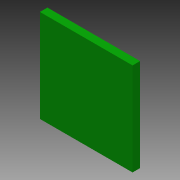
# Autodesk Inventor part: DisceepXL_PCB
Saved by Autodesk Inventor 2014 (Build 180170000, 170)
## iProperties
Created: 2014-11-22
Part Number: DisceepXL_PCB
Material: Phenolic Resin
Document SubType Name: Modeling
Designer: DV
Mass: 0.0449256 g
Surface Area: 1.26194 cm^2
Volume: 0.0325548 cm^3
Density: 1.38 g/cm^3
Appearance: Smooth - Light Orange
Author: DV
Autodesk Inventor part; units mm, degrees
ref_plane "YZ Plane" through (0, 0, 0) normal (1, 0, 0) x (0, 1, 0)
ref_plane "XZ Plane" through (0, 0, 0) normal (0, 1, 0) x (-1, 0, 0)
ref_plane "XY Plane" through (0, 0, 0) normal (0, 0, 1) x (1, 0, 0)
sketch "Sketch1" plane through (0, 0, 0) normal (0, 0, 1) x (1, 0, 0)
  line L0 (-3.683, -3.683) -> (3.683, -3.683)
  line L1 (3.683, -3.683) -> (3.683, 3.683)
  line L2 (3.683, 3.683) -> (-3.683, 3.683)
  line L3 (-3.683, 3.683) -> (-3.683, -3.683)
  point P0 (0, 0)
  dimension "d0" = 7.366
  dimension "d1" = 7.366
  dimension "d4" = 3.683
  dimension "d5" = 3.683
  constraints: 8 end point, 2 parallel, 1 horizontal, 1 perpendicular
  measures "d0" distance of L2.end L1.end
  measures "d1" distance of L1.end L0.end
  measures "d4" distance from line of L3 point (0, 0)
  measures "d5" distance from line of L0 point (0, 0)
extrude "Extrusion1" add sketch "Sketch1" along normal blind 0.6
equation "\"d4\" = 0.5 * d0"
equation "\"d5\" = d4"
body "Solid1"
